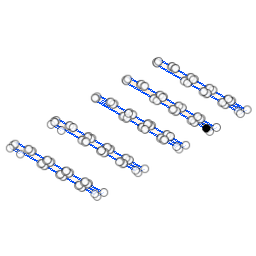
Plano_pilares v5 (Autodesk Fusion 360 design; units mm, degrees)
Autodesk Fusion 360 part; units mm, degrees
sketch "Sketch1" plane through (0, 0, 0) normal (0, 1, 0) x (1, 0, 0)
  line L0 (25, -25) -> (265, -25)
  line L1 (265, -25) -> (265, -45)
  line L2 (265, -45) -> (25, -45)
  line L3 (25, -45) -> (25, -25)
  line L4 (274.9404, -25) -> (274.9404, -33.5)
  line L5 (274.9404, -33.5) -> (274.9404, -36.5)
  line L6 (274.9404, -36.5) -> (274.9404, -45)
  line L7 (265, -33.5) -> (215, -33.5)
  line L8 (265, -36.5) -> (215, -36.5)
  line L9 (215, -33.5) -> (215, -36.5)
  line L10 (25, -25) -> (21, -25)
  line L11 (21, -32) -> (21, -38)
  line L12 (22, -31) -> (25, -31)
  line L13 (22, -39) -> (25, -39)
  arc A0 (21, -38) -> (22, -39) centre (22, -38) ccw
  arc A1 (22, -31) -> (21, -32) centre (22, -32) ccw
  line L14 (21, -25) -> (21, -28)
  line L15 (21, -28) -> (265, -28)
  line L16 (25, -45) -> (25, -42)
  line L17 (25, -45) -> (25, -42)
  line L18 (25, -42) -> (265, -42)
  line L19 (25, -50) -> (55, -50)
  line L20 (55, -45) -> (55, -42)
  line L21 (55, -42) -> (65, -42)
  line L22 (65, -42) -> (65, -45)
  line L23 (120, -42) -> (120, -45)
  line L24 (110, -45) -> (110, -42)
  line L25 (175, -42) -> (175, -45)
  line L26 (165, -45) -> (165, -42)
  line L27 (230, -42) -> (230, -45)
  line L28 (220, -45) -> (220, -42)
  line L29 (65, -25) -> (65, -28)
  line L30 (55, -28) -> (55, -25)
  line L31 (120, -25) -> (120, -28)
  line L32 (110, -28) -> (110, -25)
  line L33 (175, -25) -> (175, -28)
  line L34 (165, -28) -> (165, -25)
  line L35 (230, -25) -> (230, -28)
  line L36 (220, -28) -> (220, -25)
  line L37 (220, 75) -> (220, 78)
  line L38 (21, 92) -> (265, 92)
  line L39 (21, 88) -> (21, 82)
  line L40 (175, 78) -> (175, 75)
  line L41 (25, 75) -> (25, 78)
  line L42 (230, 95) -> (230, 92)
  line L43 (265, 95) -> (265, 75)
  line L44 (220, 92) -> (220, 95)
  line L45 (265, 75) -> (25, 75)
  line L46 (274.9404, 83.5) -> (274.9404, 75)
  line L47 (110, 92) -> (110, 95)
  line L48 (65, 95) -> (65, 92)
  line L49 (265, 83.5) -> (220, 83.5)
  line L50 (55, 75) -> (55, 78)
  line L51 (21, 95) -> (21, 92)
  line L52 (25, 75) -> (25, 78)
  line L53 (25, 78) -> (265, 78)
  line L54 (22, 89) -> (25, 89)
  line L55 (120, 78) -> (120, 75)
  line L56 (274.9404, 86.5) -> (274.9404, 83.5)
  line L57 (65, 78) -> (65, 75)
  line L58 (230, 78) -> (230, 75)
  line L59 (120, 95) -> (120, 92)
  line L60 (220, 86.5) -> (220, 83.5)
  line L61 (25, 75) -> (25, 95)
  line L62 (25, 95) -> (265, 95)
  line L63 (22, 81) -> (25, 81)
  line L64 (165, 92) -> (165, 95)
  line L65 (274.9404, 95) -> (274.9404, 86.5)
  arc A2 (21, 82) -> (22, 81) centre (22, 82) ccw
  line L66 (175, 95) -> (175, 92)
  line L67 (55, 92) -> (55, 95)
  line L68 (165, 75) -> (165, 78)
  line L69 (110, 75) -> (110, 78)
  line L70 (265, 86.5) -> (220, 86.5)
  arc A3 (22, 89) -> (21, 88) centre (22, 88) ccw
  line L71 (25, 70) -> (55, 70)
  line L72 (55, 78) -> (65, 78)
  line L73 (25, 95) -> (21, 95)
  line L74 (175, 198) -> (175, 195)
  arc A4 (21, 202) -> (22, 201) centre (22, 202) ccw
  line L75 (230, 215) -> (230, 212)
  line L76 (265, 206.5) -> (220, 206.5)
  line L77 (165, 212) -> (165, 215)
  line L78 (274.9404, 206.5) -> (274.9404, 203.5)
  line L79 (110, 212) -> (110, 215)
  line L80 (21, 215) -> (21, 212)
  line L81 (220, 206.5) -> (220, 203.5)
  line L82 (274.9404, 203.5) -> (274.9404, 195)
  line L83 (21, 208) -> (21, 202)
  line L84 (65, 215) -> (65, 212)
  line L85 (22, 209) -> (25, 209)
  line L86 (220, 212) -> (220, 215)
  line L87 (230, 198) -> (230, 195)
  line L88 (265, 203.5) -> (220, 203.5)
  line L89 (25, 215) -> (265, 215)
  line L90 (265, 215) -> (265, 195)
  line L91 (220, 195) -> (220, 198)
  line L92 (165, 195) -> (165, 198)
  line L93 (175, 215) -> (175, 212)
  line L94 (274.9404, 215) -> (274.9404, 206.5)
  arc A5 (22, 209) -> (21, 208) centre (22, 208) ccw
  line L95 (22, 201) -> (25, 201)
  line L96 (25, 195) -> (25, 198)
  line L97 (25, 195) -> (25, 198)
  line L98 (25, 215) -> (21, 215)
  line L99 (65, 198) -> (65, 195)
  line L100 (21, 212) -> (265, 212)
  line L101 (55, 198) -> (65, 198)
  line L102 (120, 198) -> (120, 195)
  line L103 (25, 198) -> (265, 198)
  line L104 (120, 215) -> (120, 212)
  line L105 (265, 195) -> (25, 195)
  line L106 (110, 195) -> (110, 198)
  line L107 (55, 195) -> (55, 198)
  line L108 (55, 212) -> (55, 215)
  line L109 (25, 195) -> (25, 215)
  line L110 (175, 288) -> (175, 285)
  line L111 (65, 288) -> (65, 285)
  line L112 (220, 302) -> (220, 305)
  line L113 (274.9404, 305) -> (274.9404, 296.5)
  line L114 (21, 298) -> (21, 292)
  line L115 (120, 288) -> (120, 285)
  line L116 (65, 305) -> (65, 302)
  line L117 (230, 305) -> (230, 302)
  line L118 (120, 305) -> (120, 302)
  line L119 (265, 285) -> (25, 285)
  line L120 (55, 288) -> (65, 288)
  line L121 (22, 291) -> (25, 291)
  line L122 (265, 296.5) -> (220, 296.5)
  arc A6 (22, 299) -> (21, 298) centre (22, 298) ccw
  line L123 (110, 285) -> (110, 288)
  line L124 (21, 302) -> (265, 302)
  line L125 (25, 305) -> (265, 305)
  line L126 (110, 302) -> (110, 305)
  line L127 (25, 288) -> (265, 288)
  line L128 (25, 305) -> (21, 305)
  line L129 (265, 305) -> (265, 285)
  line L130 (265, 293.5) -> (220, 293.5)
  line L131 (165, 285) -> (165, 288)
  line L132 (21, 305) -> (21, 302)
  line L133 (25, 285) -> (25, 288)
  line L134 (175, 305) -> (175, 302)
  line L135 (274.9404, 296.5) -> (274.9404, 293.5)
  line L136 (22, 299) -> (25, 299)
  line L137 (274.9404, 293.5) -> (274.9404, 285)
  line L138 (55, 285) -> (55, 288)
  line L139 (220, 296.5) -> (220, 293.5)
  line L140 (165, 302) -> (165, 305)
  line L141 (25, 285) -> (25, 288)
  arc A7 (21, 292) -> (22, 291) centre (22, 292) ccw
  line L142 (220, 285) -> (220, 288)
  line L143 (25, 285) -> (25, 305)
  line L144 (55, 302) -> (55, 305)
  line L145 (230, 288) -> (230, 285)
  line L146 (65, 395) -> (65, 392)
  line L147 (120, 378) -> (120, 375)
  line L148 (55, 392) -> (55, 395)
  line L149 (265, 383.5) -> (220, 383.5)
  line L150 (22, 389) -> (25, 389)
  line L151 (220, 386.5) -> (220, 383.5)
  line L152 (165, 375) -> (165, 378)
  line L153 (25, 395) -> (21, 395)
  line L154 (265, 386.5) -> (220, 386.5)
  line L155 (55, 375) -> (55, 378)
  line L156 (25, 375) -> (25, 378)
  line L157 (220, 375) -> (220, 378)
  line L158 (21, 395) -> (21, 392)
  line L159 (25, 375) -> (25, 378)
  line L160 (21, 388) -> (21, 382)
  line L161 (274.9404, 386.5) -> (274.9404, 383.5)
  line L162 (25, 375) -> (25, 395)
  line L163 (230, 395) -> (230, 392)
  line L164 (65, 378) -> (65, 375)
  line L165 (55, 378) -> (65, 378)
  line L166 (22, 381) -> (25, 381)
  arc A8 (21, 382) -> (22, 381) centre (22, 382) ccw
  arc A9 (22, 389) -> (21, 388) centre (22, 388) ccw
  line L167 (110, 375) -> (110, 378)
  line L168 (21, 392) -> (265, 392)
  line L169 (274.9404, 395) -> (274.9404, 386.5)
  line L170 (175, 395) -> (175, 392)
  line L171 (110, 392) -> (110, 395)
  line L172 (25, 378) -> (265, 378)
  line L173 (230, 378) -> (230, 375)
  line L174 (165, 392) -> (165, 395)
  line L175 (274.9404, 383.5) -> (274.9404, 375)
  line L176 (120, 395) -> (120, 392)
  line L177 (25, 395) -> (265, 395)
  line L178 (265, 375) -> (25, 375)
  line L179 (265, 395) -> (265, 375)
  line L180 (175, 378) -> (175, 375)
  line L181 (220, 392) -> (220, 395)
  line L182 (265, 392) -> (250, 392)
  line L183 (250, 392) -> (250, 390)
  line L184 (250, 390) -> (265, 390)
  line L185 (265, 390) -> (265, 392)
  line L186 (40, 208) -> (60, 208)
  line L187 (60, 208) -> (60, 202)
  line L188 (60, 202) -> (40, 202)
  line L189 (40, 202) -> (40, 208)
  dimension "d1" = 240
  dimension "d2" = 20
  dimension "d3" = 8.5
  dimension "d4" = 3
  dimension "d9" = 1
  dimension "d10" = 1
  dimension "d11" = 3
  dimension "d17" = 165
  dimension "d18" = 17
  dimension "d21" = 165
  dimension "d22" = 17
  dimension "d23" = 240
  dimension "d24" = 20
  dimension "d25" = 8.5
  dimension "d26" = 3
  dimension "d27" = 1
  dimension "d28" = 1
  dimension "d29" = 3
  dimension "d32" = 165
  dimension "d33" = 17
  dimension "d34" = 240
  dimension "d35" = 20
  dimension "d36" = 8.5
  dimension "d37" = 3
  dimension "d38" = 1
  dimension "d39" = 1
  dimension "d40" = 3
  dimension "d47" = 165
  dimension "d48" = 17
  dimension "d49" = 240
  dimension "d50" = 20
  dimension "d51" = 8.5
  dimension "d52" = 3
  dimension "d53" = 1
  dimension "d54" = 1
  dimension "d55" = 3
  dimension "d64" = 165
  dimension "d65" = 17
  dimension "d66" = 240
  dimension "d67" = 20
  dimension "d68" = 8.5
  dimension "d69" = 3
  dimension "d70" = 1
  dimension "d71" = 1
  dimension "d72" = 3
  dimension "d75" = 15
  dimension "d78" = 45
  dimension "d79" = 45
  dimension "d80" = 45
  dimension "d81" = 45
  constraint horizontal L0
  constraint vertical L1
  constraint horizontal L2
  constraint vertical L3
  constraint parallel L1 L4
  constraint parallel L4 L5
  constraint parallel L5 L6
  constraint coincident L1 L7.start
  constraint perpendicular L1 L7
  constraint coincident L1 L8.start
  constraint perpendicular L1 L8
  constraint perpendicular L7 L9
  constraint perpendicular L3 L10
  constraint perpendicular L10 L11
  constraint coincident L3 L12.end
  constraint perpendicular L11 L12
  constraint perpendicular L11 L13
  constraint tangent L11 A0
  constraint tangent L13 A0
  constraint tangent L12 A1
  constraint tangent L11 A1
  constraint perpendicular L10 L14
  constraint coincident L1 L15.end
  constraint perpendicular L1 L15
  constraint coincident L3 L16.end
  constraint perpendicular L2 L16
  constraint perpendicular L16 L18
  constraint horizontal L19
  constraint coincident L2 L20.start
  constraint coincident L18 L20.end
  constraint perpendicular L18 L20
  constraint coincident L18 L21.end
  constraint coincident L2 L22.end
  constraint perpendicular L2 L22
  constraint horizontal L62
  constraint vertical L43
  constraint horizontal L45
  constraint vertical L61
  constraint parallel L43 L65
  constraint parallel L56 L65
  constraint parallel L46 L56
  constraint coincident L70.start L43
  constraint perpendicular L43 L70
  constraint coincident L49.start L43
  constraint perpendicular L43 L49
  constraint perpendicular L60 L70
  constraint perpendicular L61 L73
  constraint perpendicular L39 L73
  constraint coincident L54.end L61
  constraint perpendicular L39 L54
  constraint perpendicular L39 L63
  constraint tangent L39 A2
  constraint tangent L63 A2
  constraint tangent L54 A3
  constraint tangent L39 A3
  constraint perpendicular L51 L73
  constraint coincident L38.end L43
  constraint perpendicular L38 L43
  constraint coincident L41.end L61
  constraint perpendicular L45 L52
  constraint perpendicular L52 L53
  constraint horizontal L71
  constraint coincident L50.start L45
  constraint coincident L50.end L53
  constraint perpendicular L50 L53
  constraint coincident L57.start L53
  constraint coincident L57.end L45
  constraint perpendicular L45 L57
  constraint horizontal L89
  constraint vertical L90
  constraint horizontal L105
  constraint vertical L109
  constraint parallel L90 L94
  constraint parallel L78 L94
  constraint parallel L78 L82
  constraint coincident L76.start L90
  constraint perpendicular L76 L90
  constraint coincident L88.start L90
  constraint perpendicular L88 L90
  constraint perpendicular L76 L81
  constraint perpendicular L98 L109
  constraint perpendicular L83 L98
  constraint coincident L85.end L109
  constraint perpendicular L83 L85
  constraint perpendicular L83 L95
  constraint tangent A4 L83
  constraint tangent A4 L95
  constraint tangent L85 A5
  constraint tangent L83 A5
  constraint perpendicular L80 L98
  constraint coincident L100.end L90
  constraint perpendicular L90 L100
  constraint coincident L96.end L109
  constraint perpendicular L96 L105
  constraint perpendicular L96 L103
  constraint coincident L107.start L105
  constraint coincident L101.start L103
  constraint perpendicular L103 L107
  constraint coincident L99.start L103
  constraint coincident L99.end L105
  constraint perpendicular L99 L105
  constraint horizontal L125
  constraint vertical L129
  constraint horizontal L119
  constraint vertical L143
  constraint parallel L113 L129
  constraint parallel L113 L135
  constraint parallel L135 L137
  constraint coincident L122.start L129
  constraint perpendicular L122 L129
  constraint coincident L130.start L129
  constraint perpendicular L129 L130
  constraint perpendicular L122 L139
  constraint perpendicular L128 L143
  constraint perpendicular L114 L128
  constraint coincident L136.end L143
  constraint perpendicular L114 L136
  constraint perpendicular L114 L121
  constraint tangent L114 A7
  constraint tangent L121 A7
  constraint tangent A6 L136
  constraint tangent L114 A6
  constraint perpendicular L128 L132
  constraint coincident L124.end L129
  constraint perpendicular L124 L129
  constraint coincident L127.start L143
  constraint perpendicular L119 L141
  constraint perpendicular L127 L141
  constraint coincident L138.start L119
  constraint coincident L120.start L127
  constraint perpendicular L127 L138
  constraint coincident L111.start L127
  constraint coincident L111.end L119
  constraint perpendicular L111 L119
  constraint horizontal L177
  constraint vertical L179
  constraint horizontal L178
  constraint vertical L162
  constraint parallel L169 L179
  constraint parallel L161 L169
  constraint parallel L161 L175
  constraint coincident L154.start L179
  constraint perpendicular L154 L179
  constraint coincident L149.start L179
  constraint perpendicular L149 L179
  constraint perpendicular L151 L154
  constraint perpendicular L153 L162
  constraint perpendicular L153 L160
  constraint coincident L150.end L162
  constraint perpendicular L150 L160
  constraint perpendicular L160 L166
  constraint tangent L160 A8
  constraint tangent L166 A8
  constraint tangent L150 A9
  constraint tangent L160 A9
  constraint perpendicular L153 L158
  constraint coincident L168.end L179
  constraint perpendicular L168 L179
  constraint coincident L156.end L162
  constraint perpendicular L156 L178
  constraint perpendicular L156 L172
  constraint coincident L155.start L178
  constraint coincident L155.end L172
  constraint perpendicular L155 L172
  constraint coincident L164.start L172
  constraint coincident L164.end L178
  constraint perpendicular L164 L178
  constraint horizontal L182
  constraint vertical L183
  constraint horizontal L184
  constraint vertical L185
  constraint horizontal L186
  constraint vertical L187
  constraint horizontal L188
  constraint vertical L189
  measures "d1" distance of L0.start L0.end
  measures "d2" distance of L0.start L2.end
  measures "d3" distance of L4.start L4.end
  measures "d4" distance of L4.end L5.end
  measures "d9" radius of A0
  measures "d10" radius of A1
  measures "d11" distance of L10.end L14.end
  measures "d23" distance of L43.start L61.end
  measures "d24" distance of L61.end L41.start
  measures "d25" distance of L56.start L65.start
  measures "d26" distance of L56.start L46.start
  measures "d27" radius of A2
  measures "d28" radius of A3
  measures "d29" distance of L51.start L38.start
  measures "d34" distance of L89.end L89.start
  measures "d35" distance of L96.start L89.start
  measures "d36" distance of L78.start L94.start
  measures "d37" distance of L78.start L78.end
  measures "d38" radius of A4
  measures "d39" radius of A5
  measures "d40" distance of L80.end L80.start
  measures "d49" distance of L125.start L125.end
  measures "d50" distance of L119.end L125.start
  measures "d51" distance of L113.end L113.start
  measures "d52" distance of L135.end L113.end
  measures "d53" radius of A7
  measures "d54" radius of A6
  measures "d55" distance of L128.end L124.start
  measures "d66" distance of L153.start L177.end
  measures "d67" distance of L156.start L153.start
  measures "d68" distance of L161.start L169.start
  measures "d69" distance of L161.end L161.start
  measures "d70" radius of A8
  measures "d71" radius of A9
  measures "d72" distance of L153.end L158.end
  measures "d75" distance of L168.end L182.end
  measures "d78" distance of L122.start L122.end
  measures "d79" distance of L149.start L149.end
  measures "d80" distance of L76.start L76.end
  measures "d81" distance of L70.start L60.start
extrude "Extrude11" add sketch "Sketch1" along normal blind 3 contours L74 L91 L103 L105 | L76 L81 L88 L90 L100 L101 L103 L109 | L92 L102 L103 L105 | L87 L90 L103 L105 | L99 L103 L105 L106 | L96 L97 L103 L105 L107 L109 | A4 L83 L85 A5 L95 L109 | L75 L86 L89 L100 | L77 L89 L93 L100 | L84 L89 L100 L108 | L79 L89 L100 L104 makes body 1
extrude "Extrude7" add sketch "Sketch1" along normal blind 3 separate body contours L146 L148 L168 L177 | L149 L151 L154 L162 L165 L168 L172 L179 L183 L184 | L168 L171 L176 L177 | L168 L170 L174 L177 | L163 L168 L177 L181 | L155 L156 L159 L162 L172 L178 | L164 L167 L172 L178 | L147 L152 L172 L178 | L157 L172 L178 L180 | L172 L173 L178 L179 makes body 2
extrude "Extrude6" add sketch "Sketch1" along normal blind 3 separate body contours L146 L148 L168 L177 | L149 L151 L154 L162 L165 L168 L172 L179 L183 L184 | L168 L171 L176 L177 | L168 L170 L174 L177 | L163 L168 L177 L181 | L155 L156 L159 L162 L172 L178 | L164 L167 L172 L178 | L147 L152 L172 L178 | L157 L172 L178 L180 | L172 L173 L178 L179 makes body 3
extrude "Extrude3" add sketch "Sketch1" along normal blind 3 separate body contours L110 L119 L127 L142 | L120 L122 L124 L127 L129 L130 L139 L143 | L115 L119 L127 L131 | L119 L127 L129 L145 | L111 L119 L123 L127 | L119 L127 L133 L138 L141 L143 | L112 L117 L124 L125 | L124 L125 L134 L140 | L116 L124 L125 L144 | L118 L124 L125 L126 makes body 4
extrude "Extrude1" add sketch "Sketch1" along normal blind 3 separate body contours L37 L40 L45 L53 | L38 L43 L49 L53 L60 L61 L70 L72 | L43 L45 L53 L58 | L45 L53 L55 L68 | L45 L53 L57 L69 | L41 L45 L50 L52 L53 L61 | L38 L42 L44 L62 | L39 L54 L61 L63 A2 A3 | L38 L62 L64 L66 | L38 L47 L59 L62 | L38 L48 L62 L67 makes body 5
extrude "Extrude2" add sketch "Sketch1" along normal blind 3 separate body contours L74 L91 L103 L105 | L76 L81 L88 L90 L100 L101 L103 L109 | L92 L102 L103 L105 | L87 L90 L103 L105 | L99 L103 L105 L106 | L96 L97 L103 L105 L107 L109 | L75 L86 L89 L100 | L77 L89 L93 L100 | L84 L89 L100 L108 | L79 L89 L100 L104 | L186 L187 L188 L189 makes body 6
copy_body "Body->Comp1" bodies 5 removing the originals makes body 7 in component "Pilar_cara_interna"
copy_body "Body->Comp2" bodies 6 removing the originals makes body 8 in component "Pilar_caras laterles "
sketch "Sketch2" plane through (0, 3, 0) normal (0, 1, 0) x (-1, 0, 0)
  line L0 (-220, -285) -> (-220, -288)
  line L1 (-220, -288) -> (-230, -288)
  line L2 (-230, -288) -> (-230, -285)
  line L3 (-230, -285) -> (-265, -285)
  line L4 (-265, -285) -> (-265, -293.5)
  line L5 (-265, -293.5) -> (-220, -293.5)
  line L6 (-220, -293.5) -> (-220, -296.5)
  line L7 (-220, -296.5) -> (-265, -296.5)
  line L8 (-265, -296.5) -> (-265, -302)
  line L9 (-265, -302) -> (-230, -302)
  line L10 (-230, -302) -> (-230, -305)
  line L11 (-230, -305) -> (-220, -305)
  line L12 (-220, -305) -> (-220, -302)
  line L13 (-220, -302) -> (-175, -302)
  line L14 (-175, -302) -> (-175, -305)
  line L15 (-175, -305) -> (-165, -305)
  line L16 (-165, -305) -> (-165, -302)
  line L17 (-165, -302) -> (-120, -302)
  line L18 (-120, -302) -> (-120, -305)
  line L19 (-120, -305) -> (-110, -305)
  line L20 (-110, -305) -> (-110, -302)
  line L21 (-110, -302) -> (-65, -302)
  line L22 (-65, -302) -> (-65, -305)
  line L23 (-65, -305) -> (-55, -305)
  line L24 (-55, -305) -> (-55, -302)
  line L25 (-55, -302) -> (-25, -302)
  line L26 (-25, -302) -> (-25, -285)
  line L27 (-25, -285) -> (-55, -285)
  line L28 (-55, -285) -> (-55, -288)
  line L29 (-55, -288) -> (-65, -288)
  line L30 (-65, -288) -> (-65, -285)
  line L31 (-65, -285) -> (-110, -285)
  line L32 (-110, -285) -> (-110, -288)
  line L33 (-110, -288) -> (-120, -288)
  line L34 (-120, -288) -> (-120, -285)
  line L35 (-120, -285) -> (-165, -285)
  line L36 (-165, -285) -> (-165, -288)
  line L37 (-165, -288) -> (-175, -288)
  line L38 (-175, -288) -> (-175, -285)
  line L39 (-175, -285) -> (-220, -285)
  line L40 (-265, -285) -> (-250, -285)
  line L41 (-250, -285) -> (-250, -290)
  line L42 (-250, -290) -> (-265, -290)
  line L43 (-265, -290) -> (-265, -285)
  dimension "d58" = 15
  dimension "d59" = 5
  constraint horizontal L40
  constraint vertical L41
  constraint horizontal L42
  constraint vertical L43
  constraint coincident L3.end L4.start
  measures "d58" distance of L3.end L40.end
  measures "d59" distance of L3.end L42.end
extrude "Extrude4" cut sketch "Sketch2" against normal blind 3 contours L3 L4 L40 L41 L42 L43 bodies 4
copy_body "Body->Comp3" bodies 3 removing the originals makes body 9 in component "Tapa_sacado1"
copy_body "Body->Comp4" bodies 4 removing the originals makes body 10 in component "Tapa_sacado2"
extrude "Extrude8" add sketch "Sketch2" along normal blind 3 separate body contours L0 L1 L2 L3 L4 L5 L6 L7 L8 L9 L10 L11 L12 L13 L14 L15 L16 L17 L18 L19 L20 L21 L22 L23 L24 L25 L26 L27 L28 L29 L30 L31 L32 L33 L34 L35 L36 L37 L38 L39 L41 L42 makes body 11
extrude "Extrude9" add sketch "Sketch1" along normal blind 3 separate body contours L74 L91 L103 L105 | L76 L81 L88 L90 L100 L101 L103 L109 | L92 L102 L103 L105 | L87 L90 L103 L105 | L99 L103 L105 L106 | L96 L97 L103 L105 L107 L109 | L75 L86 L89 L100 | L77 L89 L93 L100 | L84 L89 L100 L108 | L79 L89 L100 L104 | L186 L187 L188 L189 makes body 12
extrude "Extrude10" add sketch "Sketch1" along normal blind 3 separate body contours L37 L40 L45 L53 | L38 L43 L49 L53 L60 L61 L70 L72 | L43 L45 L53 L58 | L45 L53 L55 L68 | L45 L53 L57 L69 | L41 L45 L50 L52 L53 L61 | L38 L42 L44 L62 | L39 L54 L61 L63 A2 A3 | L38 L62 L64 L66 | L38 L47 L59 L62 | L38 L48 L62 L67 makes body 13
copy_body "Body->Comp5" bodies 2 removing the originals makes body 14 in component "Tapa_Sacado_1.2"
copy_body "Body->Comp6" bodies 11 removing the originals makes body 15 in component "Tapa_Sacado_2.2"
copy_body "Body->Comp7" bodies 12 removing the originals makes body 16 in component "Lateral_Normal"
copy_body "Body->Comp8" bodies 13 removing the originals makes body 17 in component "Interna"
copy_body "Body->Comp9" bodies 1 removing the originals makes body 18 in component "Pilar_definitivo"
component "Pilar_cara_interna" placed x (1, 0, 0) y (0, 1, 0) z (0, 0, 1) at (0, 0, 0)
component "Pilar_caras laterles " placed x (1, 0, 0) y (0, 1, 0) z (0, 0, 1) at (0, 0, 0)
component "Tapa_sacado1" placed x (1, 0, 0) y (0, 1, 0) z (0, 0, 1) at (0, 0, 0)
component "Tapa_sacado2" placed x (1, 0, 0) y (0, 1, 0) z (0, 0, 1) at (0, 0, 0)
component "Tapa_Sacado_1.2" placed x (1, 0, 0) y (0, 1, 0) z (0, 0, 1) at (0, 0, 0)
component "Tapa_Sacado_2.2" placed x (1, 0, 0) y (0, 1, 0) z (0, 0, 1) at (0, 0, 0)
component "Lateral_Normal" placed x (1, 0, 0) y (0, 1, 0) z (0, 0, 1) at (0, 0, 0)
component "Interna" placed x (1, 0, 0) y (0, 1, 0) z (0, 0, 1) at (0, 0, 0)
component "Pilar_definitivo" placed x (1, 0, 0) y (0, 1, 0) z (0, 0, 1) at (0, 0, 0)
equation "d3 = ( 17 / 2 ) * 1 mm"
equation "d25 = ( 17 / 2 ) * 1 mm"
equation "d36 = ( 17 / 2 ) * 1 mm"
equation "d51 = ( 17 / 2 ) * 1 mm"
equation "d68 = ( 17 / 2 ) * 1 mm"
named bodies: "Pilar_cara_interna", "Pilar_caras laterles", "Tapa_sacado2", "Tapa_sacado1", "Tapa_Sacado_1.2", "Tapa_Sacado_2.2", "Lateral_Normal", "Interna", "Pilar_definitivo"
